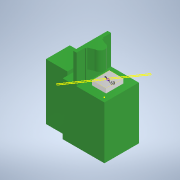
# Autodesk Inventor part: multiejes
Saved by Autodesk Inventor 2020 (Build 240168000, 168)
## iProperties
Created: 2019-10-05
Part Number: multiejes
Material: Genérico
Document SubType Name: Modeling
Designer: dasa1
Density: 1 g/cm^3
Appearance: Valor por defecto
Author: dasa1
Autodesk Inventor part; units mm, degrees
ref_plane "YZ Plane" through (0, 0, 0) normal (1, 0, 0) x (0, 1, 0)
ref_plane "XZ Plane" through (0, 0, 0) normal (0, 1, 0) x (-1, 0, 0)
ref_plane "XY Plane" through (0, 0, 0) normal (0, 0, 1) x (1, 0, 0)
sketch "Boceto1" plane through (0, 0, 0) normal (0, 1, 0) x (-1, 0, 0)
  line L0 (0, 0) -> (1225, 0)
  line L1 (1225, 0) -> (1225, -1010)
  line L2 (1225, -1010) -> (0, -1010)
  line L3 (0, -1010) -> (0, 0)
  dimension "d0" = 1225
  dimension "d1" = 1010
  constraints: 8 end point, 2 parallel, 1 horizontal, 1 perpendicular
  measures "d0" distance of L1.end L2.end
  measures "d1" distance of L0.end L1.end
extrude "Extrusión1" add sketch "Boceto1" along normal blind 1545
sketch "Boceto2" plane through (0, 0, 0) normal (0, -1, 0) x (1, 0, 0)
  line L0 (0, 0) -> (0, -1010) construction
  line L1 (-1225, 0) -> (0, 0) construction
  line L2 (-1225, -1010) -> (-1225, 0) construction
  line L3 (0, -1010) -> (-1225, -1010) construction
  line L4 (-1225, -1010) -> (-1225, 0) construction
  line L5 (-1225, 0) -> (-1225, -140) construction
  line L6 (-1225, -140) -> (-1855, -140)
  line L7 (-1855, -140) -> (-1855, -840)
  line L8 (-1855, -840) -> (-1225, -840)
  line L9 (-1225, -840) -> (-1225, -140)
  dimension "d4" = 140
  dimension "d5" = 630
  dimension "d6" = 700
  constraints: 10 end point, 2 parallel, 1 horizontal, 1 perpendicular, 1 point on line
  measures "d4" distance of L1.start L5.end
  measures "d5" distance of L8.end L7.end
  measures "d6" distance of L7.end L6.end
extrude "Extrusión2" add sketch "Boceto2" against normal blind 1649
sketch "Boceto3" plane through (0, 1545, 0) normal (0, 1, 0) x (1, 0, 0)
  line L0 (0, 0) -> (0, 1010) construction
  line L1 (0, 1010) -> (-1225, 1010) construction
  line L2 (-1225, 1010) -> (-1225, 840) construction
  line L3 (-1225, 840) -> (-1225, 140) construction
  line L4 (-1225, 140) -> (-1225, 0) construction
  line L5 (-1225, 0) -> (0, 0) construction
  line L6 (0, 1010) -> (-1225, 1010) construction
  line L7 (-1225, 1010) -> (-816.6667, 1010) construction
  line L8 (-1225, 0) -> (0, 0) projected
  line L9 (-816.6667, 1010) -> (-916.6667, 1010)
  line L10 (-916.6667, 1010) -> (-916.6667, 0)
  line L11 (-916.6667, 0) -> (-816.6667, 0)
  line L12 (-816.6667, 0) -> (-816.6667, 1010)
  point P0 (-816.6667, 0)
  dimension "d9" = 408.3333
  dimension "d10" = 100
  constraints: 10 end point, 2 parallel, 2 perpendicular, 1 horizontal, 1 point on line
  measures "d9" distance of L1.end L7.end
  measures "d10" distance of L11.end L10.end
extrude "Extrusión3" add sketch "Boceto3" along normal blind 855
sketch "Boceto4" plane through (0, 2400, 0) normal (0, 1, 0) x (1, 0, 0)
  line L0 (-916.6667, 0) -> (-816.6667, 0) construction
  line L1 (-816.6667, 0) -> (-816.6667, 1010) construction
  line L2 (-816.6667, 1010) -> (-916.6667, 1010) construction
  line L3 (-916.6667, 1010) -> (-916.6667, 0) construction
  line L4 (-916.6667, 1010) -> (-916.6667, 0) construction
  line L5 (-916.6667, 505) -> (-816.6667, 505) construction
  line L6 (-816.6667, 0) -> (-816.6667, 1010) construction
  line L7 (-816.6667, 505) -> (-816.6667, 245) construction
  line L8 (-816.6667, 245) -> (-786.6667, 245)
  line L9 (-786.6667, 245) -> (-786.6667, 765)
  line L10 (-786.6667, 765) -> (-816.6667, 765)
  line L11 (-816.6667, 765) -> (-816.6667, 245)
  point P0 (0, 0)
  dimension "d14" = 260
  dimension "d15" = 30
  dimension "d16" = 520
  constraints: 12 end point, 2 midpoint, 2 parallel, 1 horizontal, 1 perpendicular, 1 point on line
  measures "d14" distance of L5.end L7.end
  measures "d15" distance of L10.end L9.end
  measures "d16" distance of L9.end L8.end
extrude "Extrusión4" add sketch "Boceto4" against normal blind 855
sketch "Boceto5" plane through (0, 2400, 0) normal (0, 1, 0) x (1, 0, 0)
  line L0 (-916.6667, 1010) -> (-916.6667, 0) construction
  line L1 (-916.6667, 1010) -> (-916.6667, 0) construction
  line L2 (-916.6667, 0) -> (-816.6667, 0) construction
  line L3 (-816.6667, 0) -> (-816.6667, 245) construction
  line L4 (-816.6667, 245) -> (-786.6667, 245) construction
  line L5 (-786.6667, 245) -> (-786.6667, 765) construction
  line L6 (-786.6667, 765) -> (-816.6667, 765) construction
  line L7 (-816.6667, 765) -> (-816.6667, 1010) construction
  line L8 (-816.6667, 1010) -> (-916.6667, 1010) construction
  line L9 (-916.6667, 505) -> (-786.6667, 505) construction
  line L10 (-786.6667, 505) -> (-486.6667, 505) construction
  circle A0 centre (-636.6667, 505) radius 150
  line L11 (-786.6667, 765) -> (-786.6667, 245) construction
  line L12 (-548.6024, 383.5723) -> (-724.731, 383.5723) construction
  line L13 (-724.731, 383.5723) -> (-724.731, 626.4277) construction
  line L14 (-724.731, 626.4277) -> (-548.6024, 626.4277) construction
  line L15 (-548.6024, 626.4277) -> (-548.6024, 383.5723) construction
  line L16 (-786.6667, 289.3401) -> (-786.6667, 720.6599)
  line L17 (-636.6667, 355) -> (-786.6667, 289.3401)
  line L18 (-636.6667, 655) -> (-786.6667, 720.6599)
  point P0 (0, 0)
  dimension "d19" = 300
  constraints: 18 end point, 4 point on circle, 3 midpoint, 2 parallel, 2 point on line, 2 symmetric about line, 1 centre point, 1 collinear, 1 horizontal, 1 perpendicular
  measures "d19" distance of L9.end L10.end
extrude "Extrusión5" add sketch "Boceto5" against normal blind 550
sketch "Boceto6" plane through (0, 1545, 0) normal (0, 1, 0) x (1, 0, 0)
  line L0 (-786.6667, 245) -> (-816.6667, 245) construction
  line L1 (-816.6667, 245) -> (-816.6667, 0) construction
  line L2 (-816.6667, 0) -> (0, 0) construction
  line L3 (0, 0) -> (0, 1010) construction
  line L4 (0, 1010) -> (-816.6667, 1010) construction
  line L5 (-816.6667, 1010) -> (-816.6667, 765) construction
  line L6 (-816.6667, 765) -> (-786.6667, 765) construction
  line L7 (-786.6667, 765) -> (-786.6667, 245) construction
  line L8 (-816.6667, 0) -> (0, 0) construction
  line L9 (-816.6667, 0) -> (-612.4999, 0) construction
  line L10 (-816.6667, 252.5) -> (-816.6667, 0) construction
  line L11 (-204.1664, 757.5) -> (0.0003, 757.5) construction
  line L12 (0.0003, 757.5) -> (0.0003, 1010) construction
  line L13 (0.0003, 1010) -> (-204.1664, 1010) construction
  line L14 (-204.1664, 1010) -> (-204.1664, 757.5) construction
  line L15 (-816.6667, 0) -> (-612.4999, 0) construction
  line L16 (-612.4999, 0) -> (-612.4999, 252.5) construction
  line L17 (-612.4999, 252.5) -> (-816.6667, 252.5) construction
  line L18 (-816.6667, 252.5) -> (-816.6667, 0) construction
  line L19 (-612.4999, 252.5) -> (-204.1664, 252.5)
  line L20 (-204.1664, 252.5) -> (-204.1664, 757.5)
  line L21 (-204.1664, 757.5) -> (-612.4999, 757.5)
  line L22 (-612.4999, 757.5) -> (-612.4999, 252.5)
  dimension "d26" = 204.1668
  dimension "d27" = 252.5
  dimension "d28" = 204.1668
  dimension "d29" = 252.5
  constraints: 28 end point, 6 parallel, 4 horizontal, 3 perpendicular
  measures "d26" distance of L13.end L12.end
  measures "d27" distance of L12.end L11.end
  measures "d28" distance of L17.end L16.end
  measures "d29" distance of L16.end L15.end
extrude "Extrusión6" add sketch "Boceto6" along normal blind 130
sketch "Boceto7" plane through (0, 1675, 0) normal (0, 1, 0) x (1, 0, 0)
  line L0 (-204.1664, 757.5) -> (-612.4999, 757.5) construction
  line L1 (-612.4999, 757.5) -> (-612.4999, 252.5) construction
  line L2 (-612.4999, 252.5) -> (-204.1664, 252.5) construction
  line L3 (-204.1664, 252.5) -> (-204.1664, 757.5) construction
  circle A0 centre (-408.3332, 505) radius 30
  line L4 (0.369, 1326.8253) -> (-977.0627, -418.0608) projected
  line L5 (40.9134, 1306.9835) -> (-936.5183, -437.9025) projected
  point P0 (0, 0)
  dimension "d32" = 60
  constraints: 1 centre point
  measures "d32" diameter of A0
